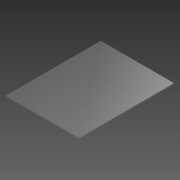
# Autodesk Inventor part: EnclosureBack
Saved by Autodesk Inventor 2015 (Build 190159000, 159)
## iProperties
Created: 2014-08-22
Part Number: EnclosureBack
Material: Polycarbonate, Clear
Document SubType Name: Modeling
Designer: t_clevj
Density: 1.2 g/cm^3
Appearance: Polycarbonate - Clear
Author: t_clevj
Autodesk Inventor part; units mm, degrees
ref_plane "YZ Plane" through (0, 0, 0) normal (1, 0, 0) x (0, 1, 0)
ref_plane "XZ Plane" through (0, 0, 0) normal (0, 1, 0) x (-1, 0, 0)
ref_plane "XY Plane" through (0, 0, 0) normal (0, 0, 1) x (1, 0, 0)
sketch "Sketch1" plane through (0, 0, 0) normal (0, 0, 1) x (1, 0, 0)
  line L0 (349, -440) -> (-1, -440) projected
  line L1 (-1, 20) -> (349, 20) projected
  line L2 (-1, 20) -> (-1, -440)
  line L3 (-1, -440) -> (349, -440)
  line L4 (349, -440) -> (349, 20)
  line L5 (349, 20) -> (-1, 20)
  point P0 (0, 0)
  constraints: 8 end point, 3 perpendicular, 1 vertical
extrude "Extrusion1" add sketch "Sketch1" along normal blind 6
sketch "Sketch2" plane through (-1, 20, 0) normal (0, 1, 0) x (1, 0, 0)
  line L0 (350, 0) -> (0, 0) projected
  line L1 (0, 0) -> (0, -6) projected
  line L2 (350, -6) -> (0, -6) projected
  line L3 (350, 0) -> (350, -6) projected
  point P0 (1, 0)
extrude "Extrusion2" add sketch "Sketch2" along normal blind 6
sketch "Sketch3" plane through (-1, -440, 0) normal (0, -1, 0) x (1, 0, 0)
  line L0 (0, 0) -> (350, 0) projected
  line L1 (350, 0) -> (350, 6) projected
  line L2 (0, 6) -> (350, 6) projected
  line L3 (0, 0) -> (0, 6) projected
  point P0 (1, 0)
extrude "Extrusion3" add sketch "Sketch3" along normal blind 6
body "Solid1"
